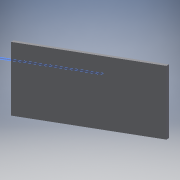
# Autodesk Inventor part: Zonnecel
Saved by Autodesk Inventor 2018.3 (Build 223284000, 284)
## iProperties
Created: 2020-11-19
Part Number: Zonnecel
Material: Generic
Document SubType Name: Modeling
Designer: daanv
Density: 1 g/cm^3
Appearance: Default
Author: daanv
Autodesk Inventor part; units mm, degrees
ref_plane "YZ Plane" through (0, 0, 0) normal (1, 0, 0) x (0, 1, 0)
ref_plane "XZ Plane" through (0, 0, 0) normal (0, 1, 0) x (-1, 0, 0)
ref_plane "XY Plane" through (0, 0, 0) normal (0, 0, 1) x (1, 0, 0)
sketch "Sketch1" plane through (0, 0, 0) normal (0, 0, 1) x (1, 0, 0)
  line L0 (0, 0) -> (0, 2)
  line L1 (0, 0) -> (72, 41.5692)
  line L2 (0, 0) -> (83.1384, 0) construction
  line L3 (72, 41.5692) -> (72, 43.5692)
  line L4 (72, 43.5692) -> (0, 2)
  dimension "d0" = 2
  dimension "d1" = 83.1384
  dimension "d2" = 30
  dimension "d3" = 2
  constraints: 10 end point, 2 vertical, 1 equal length, 1 horizontal
  measures "d0" distance of L0.start L0.end
  measures "d1" distance of L0.start L1.end
  measures "d2" angle of L2 L1
  measures "d3" distance of L1.end L3.end
extrude "Extrusion1" add sketch "Sketch1" along normal blind 50
body "Solid1"
